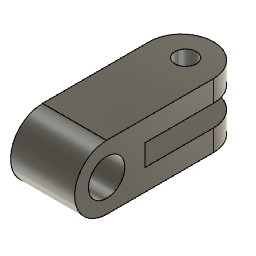
hinge 1 v2 (Autodesk Fusion 360 design; units mm, degrees)
Autodesk Fusion 360 part; units mm, degrees
note: some values were not read from the file. Set by a fixed rule: which sketch regions a step uses.
sketch "Sketch1" plane through (0, 0, 0) normal (1, 0, 0) x (0, 1, 0) in component "Component"
  circle A0 centre (-1.0944, 0.0073) radius 0.425
  line L0 (2.1063, -0.2468) -> (2.1063, -0.2424)
  line L1 (1.4084, 0.2576) -> (1.4122, 0.2576)
  line L2 (2.1063, -0.2424) -> (2.113, -0.2424)
  line L3 (-1.0958, -0.7424) -> (1.4042, -0.7424)
  line L4 (-0.1958, 0.2576) -> (1.4042, 0.2576)
  line L5 (-0.1958, 0.2576) -> (-0.1958, -0.2424)
  line L6 (-0.1958, -0.2424) -> (1.4042, -0.2424)
  line L7 (1.4042, -0.2424) -> (1.4042, -0.7424)
  line L8 (-1.0958, 0.7576) -> (1.4042, 0.7576)
  line L9 (1.4042, 0.7576) -> (1.4042, 0.2576)
  line L10 (-1.0958, 0.7576) -> (-1.0958, 0.7558)
  line L11 (-1.0958, -0.7411) -> (-1.0958, -0.7424)
  arc A1 (-1.0958, 0.7558) -> (-1.0958, -0.7411) centre (-1.0944, 0.0073) ccw
  line L12 (-2.5, -2.5) -> (0, -2.5)
  line L13 (-2.5, -2.5) -> (-2.5, -4)
  line L14 (0, -4) -> (-2.5, -4)
  circle A2 centre (0, -3.25) radius 0.25
  circle A3 centre (0, -3.25) radius 0.75
  circle A4 centre (0, -3.25) radius 0.75
  line L15 (-2.5, -2.5) -> (-2.5, -4)
  point P0 (1.4042, 0.7576)
  point P1 (-1.0958, 0.7576)
  dimension "d17" = 0.85
  dimension "d33" = 0.5
  dimension "d35" = 1.6
  dimension "d36" = 0.5
  dimension "d37" = 2.5
  dimension "d38" = 2.5
  dimension "d39" = 1.5
  dimension "d40" = 0.5
  dimension "d41" = 1.5
  constraint horizontal L3
  constraint parallel L1 L4
  constraint perpendicular L4 L5
  constraint perpendicular L5 L6
  constraint perpendicular L6 L7
  constraint horizontal L8
  constraint concentric A0 A1
  constraint coincident P0 L8.end
  constraint coincident P1 L8.start
  constraint horizontal L12
  constraint perpendicular L12 L13
  constraint concentric A2 A3
  measures "d17" diameter of A0
  measures "d33" distance of L4.start L5.end
  measures "d35" distance of L5.end L6.end
  measures "d36" distance of L6.end L3.end
  measures "d37" distance of P1 P0
  measures "d38" distance of L12.start L12.end
  measures "d39" distance of L12.start L13.end
  measures "d40" diameter of A2
  measures "d41" distance of L13.end L12.start
extrude "Extrude1" add sketch "Sketch1" along normal blind 1.5 contours L3 L4 L5 L6 L7 L8 L9 A1 in component "Component"
sketch "Sketch2" plane through (0, 0, 0.7576) normal (0, 0, 1) x (-1, 0, 0) in component "Component"
  line L0 (0, -1.4042) -> (0, 1.0958)
  line L1 (0, 1.0958) -> (-1.5, 1.0958)
  line L2 (-1.5, 1.0958) -> (-1.5, -1.4042)
  line L3 (-1.5, -1.4042) -> (0, -1.4042)
  circle A0 centre (-0.75, -1.4042) radius 0.25
  arc A1 (-1.5, -1.4042) -> (0, -1.4042) centre (-0.75, -1.4042) ccw
  dimension "d44" = 0.5
  constraint midpoint L3 A0.centre
  constraint concentric A0 A1
  constraint coincident L2 L3.start
  constraint coincident L0.start L3.end
  measures "d44" diameter of A0
extrude "Extrude2" add sketch "Sketch2" against normal blind 0.5 contours L3 A0 A1 | L3 A0 | L3 A0 in component "Component"
sketch "Sketch3" plane through (0, 0, 0.7576) normal (0, 0, 1) x (-1, 0, 0) in component "Component"
  line L0 (0, -1.4042) -> (0, 1.0958)
  line L1 (0, 1.0958) -> (-1.5, 1.0958)
  line L2 (-1.5, 1.0958) -> (-1.5, -1.4042)
  arc A0 (-1.5, -1.4042) -> (0, -1.4042) centre (-0.75, -1.4042) ccw
  circle A1 centre (-0.75, -1.5053) radius 0.25
  dimension "d47" = 0.5
  measures "d47" diameter of A1
extrude "Extrude3" cut sketch "Sketch3" against normal blind 0.5 contours A1 in component "Component"
sketch "Sketch4" plane through (0, 0, -0.7424) normal (0, 0, -1) x (1, 0, 0) in component "Component"
  line L0 (0, 1.0958) -> (0, -1.4042)
  line L1 (0, -1.4042) -> (1.5, -1.4042)
  line L2 (1.5, -1.4042) -> (1.5, 1.0958)
  line L3 (1.5, 1.0958) -> (0, 1.0958)
  circle A0 centre (0.75, -1.4042) radius 0.75
  dimension "d50" = 1.5
  constraint midpoint L1 A0.centre
  measures "d50" diameter of A0
extrude "Extrude4" add sketch "Sketch4" against normal blind 0.5 contours L1 A0 picked at (1, -1.8916) in component "Component"
component "Component" placed x (1, 0, 0) y (0, 1, 0) z (0, 0, 1) at (0, 0, 0)
